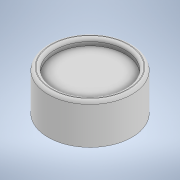
# Autodesk Inventor part: Base
Saved by Autodesk Inventor 2021 (Build 250183000, 183)
## iProperties
Created: 2024-09-30
Part Number: Base
Material: Generic
Document SubType Name: Modeling
Designer: Swoby
Density: 1 g/cm^3
Appearance: Default
Author: Swoby
Autodesk Inventor part; units mm, degrees
ref_plane "YZ Plane" through (0, 0, 0) normal (1, 0, 0) x (0, 1, 0)
ref_plane "XZ Plane" through (0, 0, 0) normal (0, 1, 0) x (-1, 0, 0)
ref_plane "XY Plane" through (0, 0, 0) normal (0, 0, 1) x (1, 0, 0)
sketch "Sketch1" plane through (0, 0, 0) normal (0, 0, 1) x (1, 0, 0)
  line L0 (0, 0) -> (0, 50)
  line L1 (0, 0) -> (62.5, 0)
  line L2 (62.5, 0) -> (62.5, 60)
  line L3 (62.5, 60) -> (52.5, 60)
  line L4 (52.5, 60) -> (52.5, 50)
  line L5 (52.5, 50) -> (0, 50)
  dimension "d0" = 125
  dimension "d1" = 60
  dimension "d2" = 50
  dimension "d3" = 10
  constraints: 12 end point, 4 perpendicular, 1 horizontal, 1 vertical
  measures "d0" diameter of L2 L0
  measures "d1" distance of L1.end L2.end
  measures "d2" distance between parallel lines of L1 L5
  measures "d3" distance of L2.end L3.end
revolve "Revolution1" add sketch "Sketch1" angle 360 about axis through (0, 0, 0) along (0, 1, 0)
fillet "Fillet1" radius 4.5 2 edges at (-62.5, 60, 0) (-52.5, 60, 0)
body "Solid1"
